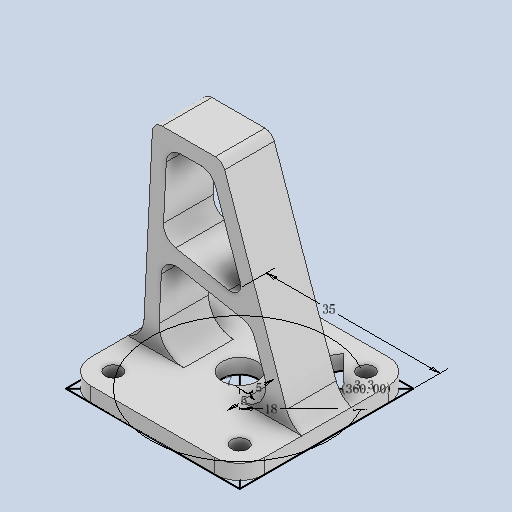
# Autodesk Inventor part: 起落架一体
Saved by Autodesk Inventor 2025.2 (Build 292293000, 293)
## iProperties
Created: 2025-10-23
Part Number: 起落架一体
Material: 常规
Document SubType Name: Modeling
Designer: BO‘S_SLAVE
Density: 1 g/cm^3
Appearance: 默认
Author: BO‘S_SLAVE
Autodesk Inventor part; units mm, degrees
ref_plane "YZ Plane" through (0, 0, 0) normal (1, 0, 0) x (0, 1, 0)
ref_plane "XZ Plane" through (0, 0, 0) normal (0, 1, 0) x (-1, 0, 0)
ref_plane "XY Plane" through (0, 0, 0) normal (0, 0, 1) x (1, 0, 0)
sketch "草图1" plane through (0, 0, 0) normal (0, 1, 0) x (-1, 0, 0)
  line L0 (0, 0) -> (35, 0)
  line L1 (35, 0) -> (35, -35)
  line L2 (35, -35) -> (0, -35)
  line L3 (0, -35) -> (0, 0)
  line L4 (0, 0) -> (35, -35)
  line L5 (35, 0) -> (0, -35)
  circle A0 centre (4.7721, -30.2279) radius 1.65
  circle A1 centre (30.2279, -30.2279) radius 1.65
  circle A2 centre (30.2279, -4.7721) radius 1.65
  circle A3 centre (4.7721, -4.7721) radius 1.65
  line L6 (0, -22.5) -> (35, -22.5)
  line L7 (0, -12.5) -> (35, -12.5)
  circle A4 centre (17.5, -17.5) radius 3.5
  line L8 (3.8516, -24.8422) -> (10.1572, -31.1479)
  line L9 (10.734, -20.8687) -> (3.8516, -24.8422)
  line L10 (14.1308, -24.2655) -> (10.734, -20.8687)
  line L11 (10.1572, -31.1479) -> (14.1308, -24.2655)
  point P0 (17.5, -17.5)
  point P1 (17.5, -17.5)
  point P2 (7.9085, -22.5)
  point P3 (12.3653, -22.5)
  dimension "d0" = 35
  dimension "d1" = 3.3
  dimension "d2" = 18
  dimension "d5" = 360
  dimension "d17" = 5
  dimension "d18" = 5
  dimension "d49" = 7
  constraints: 24 end point, 5 centre point, 5 perpendicular, 5 point on line, 2 coincident, 2 midpoint, 2 parallel, 1 horizontal, 17 other
  measures "d0" distance of L1.end L2.end
  measures "d1" diameter of A0
  measures "d2" distance of point (17.5, -17.5) A0.centre
  measures "d17" distance from line of point (17.5, -17.5) L7
  measures "d18" distance from line of point (17.5, -17.5) L6
  measures "d49" diameter of A4
extrude "拉伸1" add sketch "草图1" along normal blind 3 contours L4 A3 L7 L3 | L0 L5 A2 L7 L4 A3 | L1 L7 L5 A2 | L7 L4 A4 L5 L6 L10 L9 L3 | L1 L6 L4 A4 L5 L7 | L6 L9 L8 L5 A0 L3 | L7 L5 A4 L4 | L1 L4 A1 L6 | L5 A0 L8 L11 L10 L6 L4 A1 L2 | L9 L10 L6 | L6 L5 A4 L4 | L6 L5 L10
sketch "草图2" plane through (-35, 0, 0) normal (0, 0, 1) x (1, 0, 0)
  line L0 (0, 0) -> (35, 0) projected
  line L1 (35, 0) -> (35, 3) projected
  line L2 (0, 3) -> (35, 3) projected
  line L3 (0, 0) -> (0, 3) projected
  line L4 (35, 3) -> (0, 3) projected
  line L5 (5, 3) -> (19, 3)
  line L6 (19, 3) -> (19, 43)
  line L7 (19, 43) -> (5, 43)
  line L8 (5, 43) -> (5, 3)
  line L9 (3, 3) -> (5, 43)
  line L10 (0, 3) -> (35, 3) projected
  line L11 (33, 3) -> (19, 43)
  line L12 (33, 3) -> (19, 3)
  line L13 (5, 3) -> (3, 3)
  line L14 (29.8216, 3) -> (16.8716, 40)
  line L15 (16.8716, 40) -> (7.8537, 40)
  line L16 (7.8537, 40) -> (6.0037, 3)
  line L17 (24.8684, 17.1519) -> (6.8814, 20.5538)
  line L18 (23.724, 20.4216) -> (7.0327, 23.5784)
  point P0 (15.3783, 22)
  point P1 (29.8216, 3)
  point P2 (5, 3)
  point P3 (8, 15.6113)
  dimension "d11" = 40
  dimension "d12" = 14
  dimension "d13" = 14
  dimension "d14" = 2
  dimension "d15" = 3
  dimension "d23" = 3
  dimension "d24" = 3
  dimension "d25" = 3
  dimension "d28" = 3
  dimension "d31" = 18
  dimension "d32" = 120
  constraints: 26 end point, 9 point on line, 5 parallel, 2 collinear, 2 horizontal, 1 midpoint, 1 perpendicular
  measures "d11" distance of L5.end L6.end
  measures "d12" distance of L5.start L5.end
  measures "d13" distance of L11.start L5.end
  measures "d14" distance of L5.start L9.start
  measures "d15" distance from line of L3 L9.start
  measures "d23" distance between parallel lines of L9 L16
  measures "d24" distance between parallel lines of L7 L15
  measures "d25" distance between parallel lines of L11 L14
  measures "d28" distance between parallel lines of L18 L17
  measures "d31" distance from line of L15 point (15.378, 22)
  measures "d32" angle of L17 L14
extrude "拉伸2" add sketch "草图2" against normal up to surface (35 mm away) contours L9 L8 L2 | L2 L14 L6 L11 | L8 L7 L6 L14 L15 L16 L2 | L17 L6 L18 L14 | L16 L18 L6 L17
sketch "草图3" plane through (0, 3, 0) normal (0, 1, 0) x (1, 0, 0)
  line L0 (-35, 35) -> (0, 35)
  line L1 (0, 35) -> (0, 0)
  line L2 (0, 0) -> (-35, 0)
  line L3 (-35, 0) -> (-35, 35)
  line L4 (-35, 35) -> (0, 0)
  line L5 (0, 35) -> (-35, 0)
  circle A0 centre (-28.1066, 6.8934) radius 1.55
  circle A1 centre (-6.8934, 6.8934) radius 1.55
  circle A2 centre (-6.8934, 28.1066) radius 1.55
  circle A3 centre (-28.1066, 28.1066) radius 1.55
  line L6 (-35, 12.5) -> (0, 12.5)
  line L7 (-35, 22.5) -> (0, 22.5)
  point P0 (-17.5, 17.5)
  point P1 (-17.5, 17.5)
  point P2 (-17.5, 17.5)
  dimension "d35" = 35
  dimension "d36" = 3.1
  dimension "d37" = 15
  dimension "d38" = 360
  dimension "d39" = 5
  dimension "d40" = 5
  constraints: 16 end point, 5 perpendicular, 5 point on line, 4 centre point, 2 coincident, 2 midpoint, 2 parallel, 1 horizontal, 9 other
  measures "d35" distance of L1.end L2.end
  measures "d36" diameter of A0
  measures "d37" distance of point (-17.5, 17.5) A0.centre
  measures "d39" distance from line of point (-17.5, 17.5) L7
  measures "d40" distance from line of point (-17.5, 17.5) L6
extrude "拉伸3" cut sketch "草图3" along normal up to surface (40 mm away) contours L4 A3 L7 L3 | L0 L5 A2 L7 L4 A3 | L1 L7 L5 A2 | A3 L4 | L4 A3 | A2 L5 | L5 A2 | L6 L5 A0 L3 | L1 L4 A1 L6 | L5 A0 L6 L4 A1 L2 | A0 L5 | L5 A0 | A1 L4 | L4 A1
fillet "圆角1" radius 3 5 edges at (-18.1284, 40, -17.5) (-27.1463, 40, -17.5) (-27.9673, 23.5784, -17.5) (-10.1316, 17.1519, -17.5) (-28.1186, 20.5538, -17.5)
fillet "圆角2" radius 2 2 edges at (-16, 43, -17.5) (-30, 43, -17.5)
fillet "圆角3" radius 5 4 edges at (-5.1784, 3, -17.5) (-28.9963, 3, -17.5) (-32, 3, -17.5) (-2, 3, -17.5)
fillet "圆角4" radius 2 1 edges at (-11.276, 20.4216, -17.5)
fillet "圆角5" radius 5 4 edges at (0, 1.5, 0) (0, 1.5, -35) (-35, 1.5, -35) (-35, 1.5, 0)
